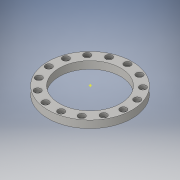
# Autodesk Inventor part: wormGearSupport
Saved by Autodesk Inventor 2016 SP1 (Build 200210100, 210)
## iProperties
Created: 2015-11-07
Part Number: wormGearSupport
Material: Generic
Document SubType Name: Modeling
Designer: steele
Density: 1 g/cm^3
Appearance: Default
Author: steele
Autodesk Inventor part; units mm, degrees
ref_plane "YZ Plane" through (0, 0, 0) normal (1, 0, 0) x (0, 1, 0)
ref_plane "XZ Plane" through (0, 0, 0) normal (0, 1, 0) x (-1, 0, 0)
ref_plane "XY Plane" through (0, 0, 0) normal (0, 0, 1) x (1, 0, 0)
sketch "Sketch1" plane through (0, 0, 0) normal (0, 1, 0) x (-1, 0, 0)
  circle A0 centre (0, 0) radius 52.9167
  circle A1 centre (0, 0) radius 72.39
  dimension "d0" = 105.8333
  dimension "d1" = 144.78
  constraints: 2 centre point, 2 coincident
  measures "d0" diameter of A0
  measures "d1" diameter of A1
extrude "Extrusion1" add sketch "Sketch1" against normal blind 12.7
sketch "Sketch2" plane through (0, 0, 0) normal (0, 1, 0) x (1, 0, 0)
  circle A0 centre (0, 64.5584) radius 2.54
  point P0 (0, 0)
  dimension "d5" = 5.08
  dimension "d6" = 64.5584
  constraints: 1 centre point
  measures "d5" diameter of A0
  measures "d6" distance of point (0, 0) A0.centre
extrude "Extrusion2" cut sketch "Sketch2" against normal through all
sketch "Sketch3" plane through (0, 0, 0) normal (0, 1, 0) x (1, 0, 0)
  circle A0 centre (0, 64.5584) radius 5.715
  point P0 (0, 0)
  dimension "d9" = 64.5584
  dimension "d10" = 11.43
  constraints: 1 centre point
  measures "d9" distance of point (0, 0) A0.centre
  measures "d10" diameter of A0
extrude "Extrusion3" cut sketch "Sketch3" against normal blind 6.35
pattern_circular "Circular Pattern3" count 15 over 360 about axis through (0, 0, 0) along (0, -1, 0) of "Extrusion2", "Extrusion3"
body "Solid1"
